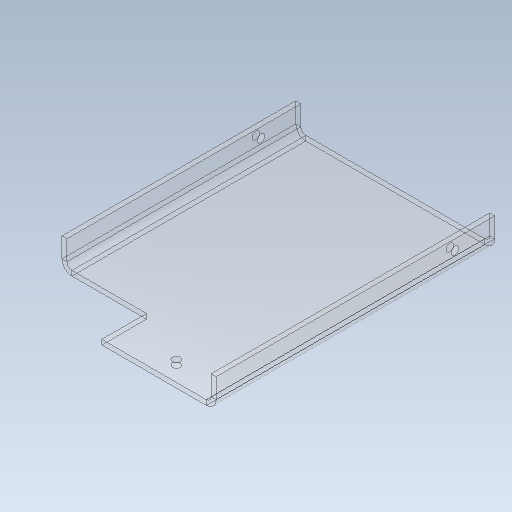
# Autodesk Inventor part: ch_frame_trayLeft
Saved by Autodesk Inventor 2020 (Build 240168000, 168)
## iProperties
Created: 2019-05-07
Part Number: ch_frame_trayLeft
Material: Polycarbonate, Clear
Document SubType Name: Sheet Metal
Designer: Victor Freire
Density: 1.2 g/cm^3
Sheet Metal Rule: Default
Appearance: Polycarbonate - Clear
Engineer: Victor Freire
Flat Pattern Width: 15.4063 cm
Flat Pattern Length: 17.78 cm
Flat Pattern Area: 273.925 cm^2
Sheet Metal Width: 6.065 in
Sheet Metal Length: 7.000 in
Sheet Metal Area: 42.458 in^2
Author: vifre
Autodesk Inventor part; units mm, degrees
ref_plane "YZ Plane" through (0, 0, 0) normal (1, 0, 0) x (0, 1, 0)
ref_plane "XZ Plane" through (0, 0, 0) normal (0, 1, 0) x (-1, 0, 0)
ref_plane "XY Plane" through (0, 0, 0) normal (0, 0, 1) x (1, 0, 0)
sketch "Sketch1" plane through (0, 0, 0) normal (0, 1, 0) x (-1, 0, 0)
  line L0 (-63.5, 88.9) -> (63.5, 88.9)
  line L1 (63.5, 88.9) -> (63.5, -88.9)
  line L2 (63.5, -88.9) -> (-63.5, -88.9)
  line L3 (-63.5, -88.9) -> (-63.5, 88.9)
  line L4 (-63.5, 88.9) -> (63.5, -88.9) construction
  line L5 (63.5, 88.9) -> (-63.5, -88.9) construction
  point P0 (0, 0)
  dimension "d0" = 177.8
  dimension "d1" = 127
extrude "Plate1" add sketch "Sketch1" along normal blind 3.175
sketch "Sketch2" plane through (0, 3.175, 0) normal (0, 1, 0) x (1, 0, 0)
  line L0 (63.5, -88.9) -> (-63.5, -88.9) projected
  line L1 (-63.5, -88.9) -> (-9.525, -88.9)
  line L2 (-9.525, -88.9) -> (-9.525, -60.325)
  line L3 (-9.525, -60.325) -> (-63.5, -60.325)
  line L4 (-63.5, -60.325) -> (-63.5, -88.9)
  point P0 (0, 0)
  dimension "d3" = 28.575
  dimension "d4" = 53.975
  constraints: 8 end point, 2 parallel, 1 horizontal, 1 perpendicular
  measures "d3" distance of L1.end L2.end
  measures "d4" distance of L2.end L3.end
extrude "Cut1" cut sketch "Sketch2" against normal blind 3.175
sketch "Sketch3" plane through (60.325, 0, -88.9) normal (1, 0, 0) x (0, 1, 0)
  line L0 (0, 177.8) -> (0, 0)
  line L1 (0, 0) -> (19.05, 0)
  line L2 (19.05, 0) -> (19.05, 177.8)
  line L3 (19.05, 177.8) -> (0, 177.8)
  constraints: 4 end point, 4 other
edge flange "Flange1" height 19.05 angle 90 thickness 3.175 bend radius 3.175 thickness toward (1, 0, 0) relief straight relief width 3.175 relief depth 1.5875 corner gap 3.175 corner form 0 edges at (63.5, 3.175, 0) (-63.5, 3.175, -14.2875) wall of the first edge with corners at (60.325, 0, 88.9) (60.325, 0, -88.9) (60.325, 19.05, -88.9) (60.325, 19.05, 88.9)
bend "Bend1"
corner "Corner1"
sketch "Sketch4" plane through (0, 3.175, 0) normal (0, 1, 0) x (1, 0, 0)
  line L0 (63.5, -88.9) -> (63.5, 88.9) projected
  line L1 (57.15, -88.9) -> (-9.525, -88.9) projected
  point P0 (0, 0)
  point P1 (25.4, -76.2)
  dimension "d24" = 38.1
  dimension "d25" = 12.7
  measures "d24" distance from line of L0 point (25.4, -76.2)
  measures "d25" distance from line of L1 point (25.4, -76.2)
hole "Hole1" at (25.4, 3.175, 76.2) direction (0, -1, 0) diameter 4.9784 end through all
sketch "Sketch5" plane through (60.325, 19.05, -88.9) normal (-1, 0, 0) x (0, 0, 1)
  line L0 (177.8, 0) -> (0, 0) projected
  line L1 (0, -12.7) -> (0, 0) projected
  point P0 (88.9, -19.05)
  point P1 (25.4, -6.35)
  dimension "d33" = 6.35
  dimension "d34" = 25.4
  measures "d33" distance from line of L0 point (25.4, -6.35)
  measures "d34" distance from line of L1 point (25.4, -6.35)
hole "Hole2" at (60.325, 12.7, -63.5) direction (1, 0, 0) diameter 4.9784 end through all
sketch "Sketch6" plane through (-60.325, 19.05, 60.325) normal (1, 0, 0) x (0, 0, -1)
  line L0 (149.225, 0) -> (0, 0) projected
  line L1 (149.225, -12.7) -> (149.225, 0) projected
  point P0 (60.325, -19.05)
  point P1 (123.825, -6.35)
  dimension "d42" = 6.35
  dimension "d43" = 25.4
  measures "d42" distance from line of L0 point (123.825, -6.35)
  measures "d43" distance from line of L1 point (123.825, -6.35)
hole "Hole3" at (-60.325, 12.7, -63.5) direction (-1, 0, 0) diameter 4.9784 end through all
equation "\"d5\" = Thickness"
equation "\"d22\" = Thickness"
equation "\"d31\" = Thickness"
equation "\"d40\" = Thickness"
equation "\"d2\" = Thickness"
equation "\"d7\" = BendReliefWidth"
equation "\"d8\" = BendReliefDepth"
equation "\"d9\" = MinimumRemnant"
equation "\"d10\" = TransitionRadius"
equation "\"d13\" = BendRadius"
equation "\"d14\" = CornerReliefSize"
equation "\"d15\" = GapSize"
equation "\"d16\" = JacobiRadiusSize"
equation "\"BendRadius\" = Thickness"
equation "\"BendReliefWidth\" = Thickness"
equation "\"BendReliefDepth\" = 0.5 * Thickness"
equation "\"CornerReliefSize\" = 4 * Thickness"
equation "\"MinimumRemnant\" = 2 * Thickness"
equation "\"TransitionRadius\" = BendRadius"
equation "\"JacobiRadiusSize\" = BendRadius"
equation "\"GapSize\" = Thickness"
equation "\"Thickness\" = 3.175"
body "Solid1"
